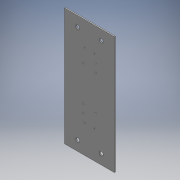
# Autodesk Inventor part: bottom_board
Saved by Autodesk Inventor 2016 (Build 200138000, 138)
## iProperties
Created: 2016-11-05
Part Number: bottom_board
Material: 一般
Document SubType Name: Modeling
Designer: 宏太
Density: 1 g/cm^3
Appearance: 既定
Mass: 41.2921 g
Surface Area: 428.281 cm^2
Volume: 41.2921 cm^3
Author: 宏太
Autodesk Inventor part; units mm, degrees
ref_plane "YZ Plane" through (0, 0, 0) normal (1, 0, 0) x (0, 1, 0)
ref_plane "XZ Plane" through (0, 0, 0) normal (0, 1, 0) x (-1, 0, 0)
ref_plane "XY Plane" through (0, 0, 0) normal (0, 0, 1) x (1, 0, 0)
sketch "スケッチ1" plane through (0, 0, 0) normal (0, 1, 0) x (-1, 0, 0)
  line L0 (0, 0) -> (110, 0)
  line L1 (110, 0) -> (110, -260)
  line L2 (110, -260) -> (0, -260)
  line L3 (0, -260) -> (0, 0)
  dimension "d0" = 110
  dimension "d1" = 260
  constraints: 8 end point, 2 parallel, 1 horizontal, 1 perpendicular
  measures "d0" distance of L1.end L2.end
  measures "d1" distance of L0.end L1.end
extrude "押し出し1" add sketch "スケッチ1" along normal blind 2
sketch "スケッチ2" plane through (0, 0, 0) normal (0, -1, 0) x (1, 0, 0)
  line L0 (0, -260) -> (0, 0) projected
  line L1 (0, 0) -> (-110, 0) projected
  line L2 (-110, -260) -> (0, -260) projected
  circle A0 centre (-41.5, -72) radius 1.1
  circle A1 centre (-41.5, -90) radius 1.1
  circle A2 centre (-68.5, -85) radius 1.1
  circle A3 centre (-66, -54.5) radius 1.1
  circle A4 centre (-44, -54.5) radius 1.1
  circle A5 centre (-44, -197.5) radius 1.1
  circle A6 centre (-66, -197.5) radius 1.1
  circle A7 centre (-68.5, -180) radius 1.1
  circle A8 centre (-68.5, -162) radius 1.1
  circle A9 centre (-41.5, -167) radius 1.1
  circle A10 centre (-29, -22) radius 4.2
  circle A11 centre (-81, -22) radius 4.2
  line L3 (-110, 0) -> (-110, -260) projected
  circle A12 centre (-81, -238) radius 4.2
  circle A13 centre (-29, -238) radius 4.2
  dimension "d30" = 2.2
  dimension "d32" = 72
  dimension "d33" = 2.2
  dimension "d35" = 2.2
  dimension "d37" = 85
  dimension "d40" = 41.5
  dimension "d41" = 41.5
  dimension "d42" = 2.2
  dimension "d44" = 54.5
  dimension "d45" = 2.2
  dimension "d47" = 54.5
  dimension "d48" = 66
  dimension "d49" = 44
  dimension "d57" = 90
  dimension "d58" = 2.2
  dimension "d59" = 44
  dimension "d60" = 197.5
  dimension "d61" = 2.2
  dimension "d62" = 66
  dimension "d63" = 197.5
  dimension "d64" = 2.2
  dimension "d65" = 68.5
  dimension "d66" = 180
  dimension "d67" = 2.2
  dimension "d68" = 68.5
  dimension "d69" = 162
  dimension "d70" = 2.2
  dimension "d71" = 41.5
  dimension "d72" = 167
  dimension "d75" = 8.4
  dimension "d76" = 29
  dimension "d77" = 22
  dimension "d78" = 8.4
  dimension "d79" = 29
  dimension "d80" = 22
  dimension "d81" = 68.5
  dimension "d82" = 8.4
  dimension "d83" = 29
  dimension "d84" = 22
  dimension "d85" = 8.4
  dimension "d86" = 29
  dimension "d87" = 22
  constraints: 14 centre point
  measures "d30" diameter of A0
  measures "d32" distance from line of L1 A0.centre
  measures "d33" diameter of A1
  measures "d35" diameter of A2
  measures "d37" distance from line of L1 A2.centre
  measures "d40" distance from line of L0 A1.centre
  measures "d41" distance from line of L0 A0.centre
  measures "d42" diameter of A3
  measures "d44" distance from line of L1 A3.centre
  measures "d45" diameter of A4
  measures "d47" distance from line of L1 A4.centre
  measures "d48" distance from line of L0 A3.centre
  measures "d49" distance from line of L0 A4.centre
  measures "d57" distance from line of L1 A1.centre
  measures "d58" diameter of A5
  measures "d59" distance from line of L0 A5.centre
  measures "d60" distance from line of L1 A5.centre
  measures "d61" diameter of A6
  measures "d62" distance from line of L0 A6.centre
  measures "d63" distance from line of L1 A6.centre
  measures "d64" diameter of A7
  measures "d65" distance from line of L0 A7.centre
  measures "d66" distance from line of L1 A7.centre
  measures "d67" diameter of A8
  measures "d68" distance from line of L0 A8.centre
  measures "d69" distance from line of L1 A8.centre
  measures "d70" diameter of A9
  measures "d71" distance from line of L0 A9.centre
  measures "d72" distance from line of L1 A9.centre
  measures "d75" diameter of A10
  measures "d76" distance from line of L0 A10.centre
  measures "d77" distance from line of A10.centre L1
  measures "d78" diameter of A11
  measures "d79" distance from line of A11.centre L3
  measures "d80" distance from line of A11.centre L1
  measures "d81" distance from line of A2.centre L0
  measures "d82" diameter of A12
  measures "d83" distance from line of A12.centre L3
  measures "d84" distance from line of L2 A12.centre
  measures "d85" diameter of A13
  measures "d86" distance from line of L0 A13.centre
  measures "d87" distance from line of L2 A13.centre
extrude "押し出し7" cut sketch "スケッチ2" against normal blind 2 contours A0 | A1 | A2 | A3 | A4 | A5 | A6 | A7 | A8 | A9 | A10 | A11 | A12 | A13
